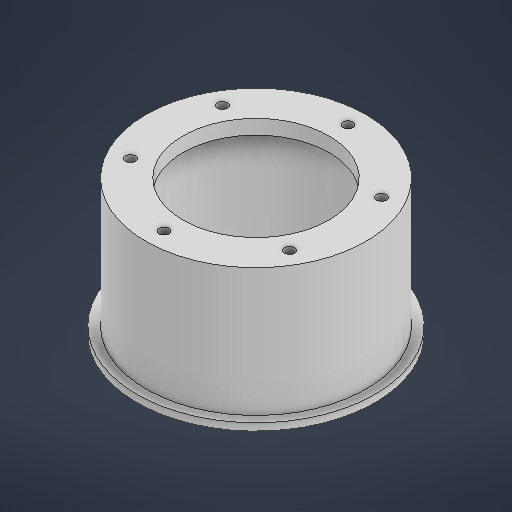
# Autodesk Inventor part: Cylinder Replacement- 11
Saved by Autodesk Inventor 2025 (Build 290162000, 162)
## iProperties
Created: 2024-04-11
Part Number: Cylinder Replacement- 11
Material: Generic
Document SubType Name: Modeling
Designer: Thienan Hoang
Density: 1 g/cm^3
Appearance: Default
Author: Thienan Hoang
Autodesk Inventor part; units mm, degrees
ref_plane "YZ Plane" through (0, 0, 0) normal (1, 0, 0) x (0, 1, 0)
ref_plane "XZ Plane" through (0, 0, 0) normal (0, 1, 0) x (-1, 0, 0)
sketch "Sketch1" plane through (0, 0, 0) normal (0, 1, 0) x (-1, 0, 0)
  circle A0 centre (0, 0) radius 66
  circle A1 centre (0, 0) radius 61
  circle A2 centre (0, 0) radius 59
  dimension "Absolute_Diameter" = 132
  dimension "Diameter_No_Outer_Lip" = 122
  dimension "Inner_Cylinder_Diameter" = 118
  constraints: 3 centre point, 3 coincident
  measures "Absolute_Diameter" diameter of A0
  measures "Diameter_No_Outer_Lip" diameter of A1
  measures "Inner_Cylinder_Diameter" diameter of A2
extrude "Extrusion1" add sketch "Sketch1" along normal blind 4 contours A0
extrude "Extrusion2" add sketch "Sketch1" along normal blind 75 contours A1
sketch "Sketch2" plane through (0, 75, 0) normal (0, 1, 0) x (1, 0, 0)
  circle A0 centre (0, 0) radius 40.5
  circle A1 centre (0, 0) radius 61
  dimension "Lip_Diameter_Out" = 81
  dimension "Top_Outer_Lip_Diameter" = 122
  constraints: 2 centre point, 2 coincident
  measures "Lip_Diameter_Out" diameter of A0
  measures "Top_Outer_Lip_Diameter" diameter of A1
extrude "Extrusion7" add sketch "Sketch2" against normal blind 8
ref_plane "Work Plane2" through (0, 10, 0) normal (0, 1, 0) x (1, 0, 0)
sketch "Sketch3" plane through (0, 10, 0) normal (0, 1, 0) x (1, 0, 0)
  circle A0 centre (0, 0) radius 127.5
  circle A1 centre (-127.5, 0) radius 2.5
  circle A2 centre (-103.1497, -74.9426) radius 2.5
  circle A3 centre (-39.3997, -121.2597) radius 2.5
  circle A4 centre (39.3997, -121.2597) radius 2.5
  circle A5 centre (103.1497, -74.9426) radius 2.5
  circle A6 centre (127.5, 0) radius 2.5
  circle A7 centre (103.1497, 74.9426) radius 2.5
  circle A8 centre (39.3997, 121.2597) radius 2.5
  circle A9 centre (-39.3997, 121.2597) radius 2.5
  circle A10 centre (-103.1497, 74.9426) radius 2.5
  dimension "d27" = 255
  dimension "d28" = 5
  dimension "d31" = 360
  constraints: 10 centre point, 1 coincident, 1 horizontal alignment, 23 other
  measures "d28" diameter of A1
extrude "Extrusion8" [suppressed]
sketch "Sketch24" plane through (0, 75, 0) normal (0, 1, 0) x (1, 0, 0)
  circle A0 centre (0, 0) radius 51
  circle A1 centre (0, -51) radius 2.75
  circle A2 centre (44.1673, -25.5) radius 2.75
  circle A3 centre (44.1673, 25.5) radius 2.75
  circle A4 centre (0, 51) radius 2.75
  circle A5 centre (-44.1673, 25.5) radius 2.75
  circle A6 centre (-44.1673, -25.5) radius 2.75
  dimension "d230" = 102
  dimension "d231" = 5.5
  dimension "d234" = 360
  constraints: 6 centre point, 1 coincident, 1 vertical alignment, 15 other
  measures "d231" diameter of A1
extrude "Extrusion30" cut sketch "Sketch24" against normal blind 10 contours A3 A0 | A0 A3 | A2 A0 | A0 A2 | A4 A0 | A0 A4 | A1 A0 | A0 A1 | A5 A0 | A0 A5 | A6 A0 | A0 A6
body "Solid1"
